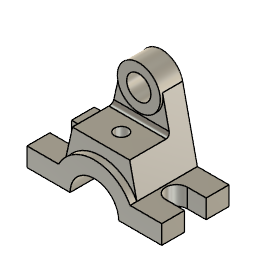
47 (Autodesk Fusion 360 design; units mm, degrees)
Autodesk Fusion 360 part; units mm, degrees
sketch "草图1" plane through (0, 0, 0) normal (0, 1, 0) x (1, 0, 0)
  line L0 (-100, 0) -> (100, 0) construction
  line L1 (-50, 0) -> (-50, -14)
  line L2 (-50, -14) -> (-26.533, -14)
  arc A0 (-26.533, -14) -> (26.533, -14) centre (0, 0) ccw
  line L3 (26.533, -14) -> (50, -14)
  line L4 (50, -14) -> (50, 0)
  line L5 (18, 0) -> (50, 0)
  line L6 (-50, 0) -> (-18, 0)
  line L7 (0, -85) -> (0, 30) construction
  arc A1 (-18, 0) -> (18, 0) centre (0, 0) ccw
  circle A2 centre (0, -60) radius 16
  circle A3 centre (0, -60) radius 9
  line L8 (-26.533, -14) -> (-15.6243, -63.4469)
  line L9 (26.533, -14) -> (15.6243, -63.4469)
  line L10 (-21.2383, -38) -> (21.2383, -38)
  dimension "d1" = 14
  dimension "d2" = 14
  dimension "d3" = 100
  dimension "d5" = 30
  dimension "d6" = 18
  dimension "d7" = 32
  dimension "d8" = 18
  dimension "d9" = 60
  dimension "d10" = 38
  constraint horizontal L0
  constraint coincident L0 L1.start
  constraint perpendicular L0 L1
  constraint perpendicular L1 L2
  constraint horizontal L3
  constraint coincident L0 L4.end
  constraint perpendicular L0 L4
  constraint coincident L0 L5.start
  constraint coincident L0 L6.end
  constraint symmetric L1 L4 L7
  constraint coincident A0.centre A1.centre
  constraint coincident L7 A2.centre
  constraint concentric A2 A3
  constraint coincident A2 L8.end
  constraint tangent A2 L8
  constraint coincident A2 L9.end
  constraint tangent A2 L9
  constraint coincident L8 L10.start
  constraint coincident L9 L10.end
  constraint horizontal L10
  measures "d1" distance of L3.end L4.end
  measures "d2" distance of L1.start L1.end
  measures "d3" distance of L1.start L4.end
  measures "d5" radius of A0
  measures "d6" radius of A1
  measures "d7" diameter of A2
  measures "d8" diameter of A3
  measures "d9" distance of A0.centre A2.centre
  measures "d10" distance of A0.centre L10
extrude "拉伸1" add sketch "草图1" against normal blind 50 contours L1 L2 A0 L3 L4 L5 L6 A1 makes body 1
extrude "拉伸2" add sketch "草图1" against normal blind 45 contours A0 L8 L9 L10 bodies 1
extrude "拉伸3" add sketch "草图1" against normal blind 15 contours A2 L8 L9 L10 bodies 1
extrude "拉伸4" add sketch "草图1" against normal blind 17 contours A2 bodies 1
sketch "草图2" plane through (0, 0, 0) normal (1, 0, 0) x (0, 1, 0)
  line L0 (-15, 63.4469) -> (-15, 41)
  line L1 (-18, 38) -> (-45, 38)
  arc A0 (-18, 38) -> (-15, 41) centre (-18, 41) ccw
  line L2 (-15, 63.4469) -> (-15, 38)
  line L3 (-15, 38) -> (-45, 38)
  point P0 (-15, 63.4469)
  point P1 (-45, 38)
  point P2 (-15, 38)
  dimension "d19" = 3
  constraint coincident P0 L0.start
  constraint coincident P1 L1.end
  constraint tangent L0 A0
  constraint tangent L1 A0
  constraint coincident P2 L2.end
  measures "d19" radius of A0
extrude "拉伸5" add sketch "草图2" along normal mid plane 54 separate body makes body 2
extrude "拉伸6" cut sketch "草图1" against normal blind 75 contours A2 L8 L9 L10 keep common part bodies 2
combine "合并1" operation add target body 1 tool bodies 2
sketch "草图3" plane through (0, 0, 0) normal (0, 0, 1) x (1, 0, 0)
  line L0 (-50, -17) -> (-50, -33)
  line L1 (-50, -33) -> (-36, -33)
  arc A0 (-36, -33) -> (-36, -17) centre (-36, -25) ccw
  line L2 (-36, -17) -> (-50, -17)
  line L3 (0, 15) -> (0, -36) construction
  line L4 (36, -17) -> (50, -17)
  line L5 (50, -17) -> (50, -33)
  line L6 (50, -33) -> (36, -33)
  arc A1 (36, -17) -> (36, -33) centre (36, -25) ccw
  dimension "d24" = 50
  dimension "d25" = 36
  dimension "d26" = 16
  dimension "d27" = 25
  constraint vertical L0
  constraint perpendicular L0 L1
  constraint tangent L1 A0
  constraint perpendicular L0 L2
  constraint vertical L3
  constraint tangent A0 L2
  constraint symmetric L0.start L3 L4.end
  constraint symmetric L0.end L3 L5.end
  constraint symmetric L1.end L3 L6.end
  constraint symmetric A0.end L3 L4.start
  constraint symmetric A0 L3 A1
  measures "d24" distance of origin L0
  measures "d25" horizontal distance of origin A0.centre
  measures "d26" distance of L0.start L0.end
  measures "d27" vertical distance of origin A0.centre
extrude "拉伸7" cut sketch "草图3" along normal blind 14 bodies 1
sketch "草图4" plane through (0, 0, 38) normal (0, 0, 1) x (-1, 0, 0)
  line L0 (-21.2383, 18) -> (21.2383, 18)
  line L1 (21.2383, 18) -> (21.2383, 45)
  line L2 (21.2383, 45) -> (-21.2383, 45)
  line L3 (-21.2383, 45) -> (-21.2383, 18)
  circle A0 centre (0, 30) radius 5
  line L4 (0, 45) -> (0, 18) construction
  dimension "d30" = 15
  dimension "d31" = 10
  constraint midpoint L2 L4.start
  constraint midpoint L0 L4.end
  constraint collinear A0.centre L4.start L4.end
  measures "d30" distance of L2 A0.centre
  measures "d31" diameter of A0
extrude "拉伸8" cut sketch "草图4" against normal blind 57 contours A0 bodies 1
equation "d10 = 60 mm - 22 mm"
